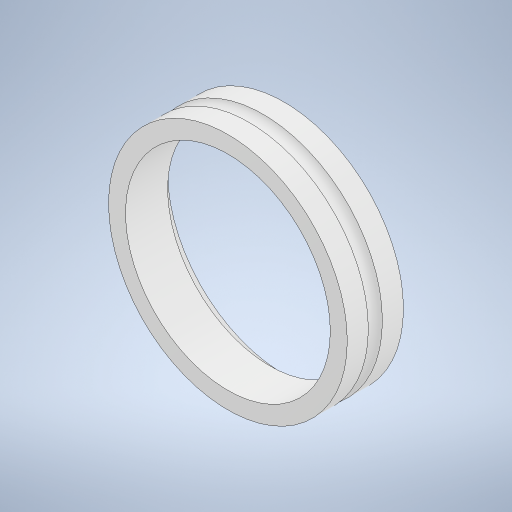
# Autodesk Inventor part: Ring Hub
Saved by Autodesk Inventor 2023.2 (Build 272271000, 271)
## iProperties
Created: 2023-06-11
Part Number: Ring Hub
Material: Nylon 6/6
Document SubType Name: Modeling
Designer: Nathan Cai
Mass: 7.80815 g
Surface Area: 49.5228 cm^2
Volume: 6.90987 cm^3
Density: 1.13 g/cm^3
Appearance: Smooth - White
Author: Nathan Cai
Autodesk Inventor part; units mm, degrees
ref_plane "YZ Plane" through (0, 0, 0) normal (1, 0, 0) x (0, 1, 0)
ref_plane "XZ Plane" through (0, 0, 0) normal (0, 1, 0) x (-1, 0, 0)
ref_plane "XY Plane" through (0, 0, 0) normal (0, 0, 1) x (1, 0, 0)
sketch "Sketch1" plane through (0, 0, 0) normal (0, 0, 1) x (1, 0, 0)
  circle A0 centre (0, 0) radius 23.15
  circle A1 centre (0, 0) radius 26.9875
  dimension "d0" = 46.3
  dimension "d1" = 53.975
  constraints: 2 centre point, 2 coincident
  measures "d0" diameter of A0
  measures "d1" diameter of A1
extrude "Extrusion1" add sketch "Sketch1" along normal blind 12.7
chamfer "Chamfer1" distance 3.175 angle 45 1 edges at (-23.15, 0, 0)
sketch "Sketch2" plane through (0, 0, 0) normal (1, 0, 0) x (0, 1, 0)
  line L0 (26.9875, 0) -> (26.9875, 12.7) projected
  circle A0 centre (26.9875, 6.35) radius 1.5875
  line L1 (0, 0) -> (0, 25.7479) construction
  dimension "d7" = 3.175
  constraints: 2 end point, 1 centre point, 1 midpoint, 1 vertical
  measures "d7" diameter of A0
revolve "Revolution1" cut sketch "Sketch2" angle 360 about axis through (0, 0, 0) along (0, 0, 1)
body "Solid1"
